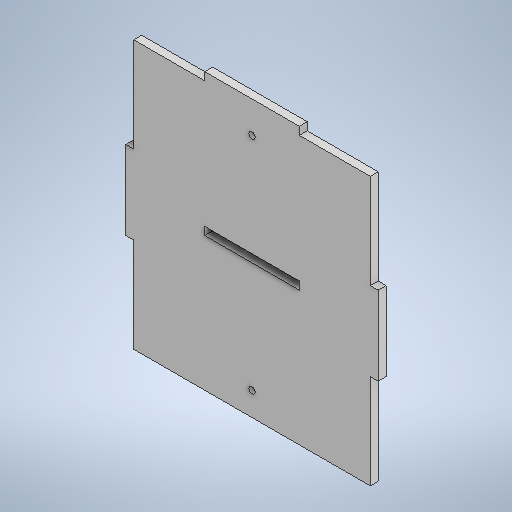
# Autodesk Inventor part: back
Saved by Autodesk Inventor 2025.3 (Build 293356030, 356C)
## iProperties
Created: 2026-06-26
Part Number: back
Material: Generic
Document SubType Name: Modeling
Designer: user
Density: 1 g/cm^3
Appearance: Default
Author: user
Autodesk Inventor part; units mm, degrees
ref_plane "YZ Plane" through (0, 0, 0) normal (1, 0, 0) x (0, 1, 0)
ref_plane "XZ Plane" through (0, 0, 0) normal (0, 1, 0) x (-1, 0, 0)
ref_plane "XY Plane" through (0, 0, 0) normal (0, 0, 1) x (1, 0, 0)
sketch "Sketch1" plane through (0, 0, 0) normal (0, 0, 1) x (1, 0, 0)
  line L0 (0, 0) -> (150, 0)
  line L1 (150, 0) -> (150, 170)
  line L2 (150, 170) -> (0, 170)
  line L3 (0, 170) -> (0, 0)
  line L4 (0, 60) -> (-5, 60)
  line L5 (-5, 60) -> (-5, 110)
  line L6 (-5, 110) -> (0, 110)
  line L7 (0, 110) -> (0, 60)
  line L8 (75, 0) -> (75, 170) construction
  line L9 (150, 60) -> (155, 60)
  line L10 (155, 60) -> (155, 110)
  line L11 (155, 110) -> (150, 110)
  line L12 (150, 110) -> (150, 60)
  line L13 (45, 85) -> (105, 85)
  line L14 (105, 85) -> (105, 90)
  line L15 (105, 90) -> (45, 90)
  line L16 (45, 90) -> (45, 85)
  line L17 (0, 85) -> (150, 85) construction
  line L18 (45, 170) -> (105, 170)
  line L19 (105, 170) -> (105, 175)
  line L20 (105, 175) -> (45, 175)
  line L21 (45, 175) -> (45, 170)
  point P0 (0, 110)
  point P1 (10, 0)
  point P2 (45, 87.5)
  dimension "d0" = 150
  dimension "d1" = 170
  dimension "d2" = 5
  dimension "d3" = 50
  dimension "d6" = 60
  dimension "d7" = 5
  dimension "d13" = 80
  dimension "d14" = 30
  dimension "d30" = 60
  dimension "d31" = 5
  dimension "d32" = 45
  dimension "d44" = 60
  constraints: 44 end point, 8 parallel, 5 midpoint, 4 horizontal, 4 perpendicular, 4 symmetric about line, 3 point on line
  measures "d0" distance of L2.end L1.end
  measures "d1" distance of L1.end L0.end
  measures "d2" distance of L5.end L6.end
  measures "d3" distance of L4.end L5.end
  measures "d6" distance of L15.end L14.end
  measures "d7" distance of L14.end L13.end
  measures "d13" distance between parallel lines of L2 L15
  measures "d14" distance from line of point (45, 87.5) L8
  measures "d30" distance of L20.end L19.end
  measures "d31" distance of L19.end L18.end
  measures "d32" distance between parallel lines of L1 L19
  measures "d44" distance between parallel lines of L0 L4
extrude "Extrusion1" add sketch "Sketch1" along normal blind 5
sketch "Sketch2" plane through (0, 0, 5) normal (0, 0, 1) x (1, 0, 0)
  line L0 (150, 170) -> (0, 170) projected
  line L1 (0, 0) -> (150, 0) projected
  line L2 (0, 170) -> (0, 110) projected
  line L3 (0, 60) -> (0, 0) projected
  point P0 (75, 15)
  dimension "d24" = 15
  dimension "d29" = 75
  measures "d24" distance from line of L1 point (75, 15)
  measures "d29" distance from line of L3 point (75, 15)
hole "Hole1" at (75, 15, 5) direction (0, 0, -1) diameter 4 end through all
sketch "Sketch3" plane through (0, 0, 5) normal (0, 0, 1) x (1, 0, 0)
  line L0 (105, 175) -> (45, 175) projected
  line L1 (45, 175) -> (45, 170) projected
  line L2 (0, 170) -> (0, 110) projected
  point P0 (0, 0)
  point P1 (75, 155)
  dimension "d40" = 20
  dimension "d45" = 75
  measures "d40" distance from line of point (75, 155) L0
  measures "d45" distance from line of L2 point (75, 155)
hole "Hole2" at (75, 155, 5) direction (0, 0, -1) diameter 4 end through all
body "Solid1"
